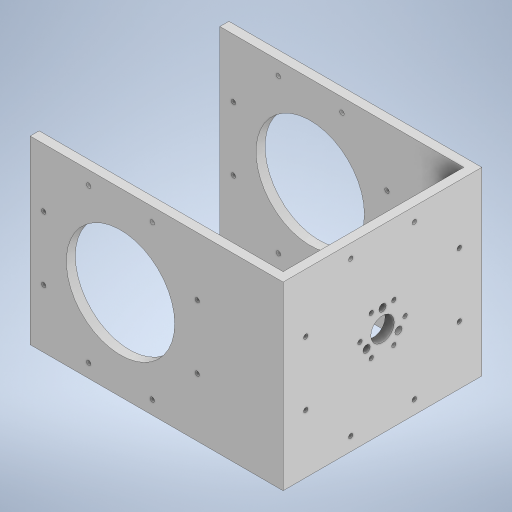
# Autodesk Inventor part: legparts_07(three)
Saved by Autodesk Inventor 2024.3 (Build 283343000, 343)
## iProperties
Created: 2024-10-21
Part Number: legparts_07(three)
Material: 一般
Document SubType Name: Modeling
Designer: 佐藤智貴
Density: 1 g/cm^3
Appearance: 既定
Mass: 104.488 g
Surface Area: 473.803 cm^2
Volume: 104.488 cm^3
Author: 佐藤智貴
Autodesk Inventor part; units mm, degrees
ref_plane "YZ Plane" through (0, 0, 0) normal (1, 0, 0) x (0, 1, 0)
ref_plane "XZ Plane" through (0, 0, 0) normal (0, 1, 0) x (-1, 0, 0)
ref_plane "XY Plane" through (0, 0, 0) normal (0, 0, 1) x (1, 0, 0)
sketch "スケッチ1" plane through (0, 0, 0) normal (0, 0, 1) x (1, 0, 0)
  circle A0 centre (0, 0) radius 48.5
  circle A1 centre (0, 0) radius 46.0893
  line L0 (-50, 50) -> (50, 50)
  line L1 (50, 50) -> (50, -50)
  line L2 (50, -50) -> (-50, -50)
  line L3 (-50, -50) -> (-50, 50)
  dimension "d0" = 97
  dimension "d3" = 50
  dimension "d4" = 50
  dimension "d5" = 50
  dimension "d6" = 50
  constraints: 8 end point, 2 centre point, 2 parallel, 1 coincident, 1 horizontal, 1 perpendicular
  measures "d0" diameter of A0
  measures "d3" distance from line of L0 point (0, 0)
  measures "d4" distance from line of L2 point (0, 0)
  measures "d5" distance from line of L1 point (0, 0)
  measures "d6" distance from line of point (0, 0) L3
extrude "押し出し1" add sketch "スケッチ1" along normal blind 5 contours A0 | A1 | L0 L1 L2 L3
sketch "スケッチ2" plane through (0, 0, 5) normal (0, 0, 1) x (1, 0, 0)
  circle A0 centre (0, 0) radius 46
  line L0 (0, 0) -> (0, 64.6511)
  line L1 (0, 0) -> (-25.9524, 62.6547)
  line L2 (-50, 50) -> (-50, -50) projected
  point P0 (-17.6034, 42.4985)
  point P1 (-42.4985, 17.6034)
  point P2 (-42.4985, -17.6034)
  point P3 (-17.6034, -42.4985)
  point P4 (17.6034, -42.4985)
  point P5 (42.4985, -17.6034)
  point P6 (42.4985, 17.6034)
  point P7 (17.6034, 42.4985)
  dimension "d7" = 92
  dimension "d8" = 22.5
  dimension "d11" = 360
  dimension "d76" = 50
  constraints: 4 end point, 1 coincident, 1 point on line, 1 vertical, 12 other
  measures "d8" angle of L0 L1
  measures "d76" distance from line of L2 point (0, 0)
hole "穴1" at (-17.6034, 42.4985, 5) at (-42.4985, 17.6034, 5) at (-42.4985, -17.6034, 5) at (-17.6034, -42.4985, 5) at (17.6034, -42.4985, 5) at (42.4985, -17.6034, 5) at (42.4985, 17.6034, 5) at (17.6034, 42.4985, 5) direction (0, 0, -1) diameter 2.459 end through all
sketch "スケッチ3" plane through (0, 0, 5) normal (0, 0, 1) x (1, 0, 0)
  circle A0 centre (0, 0) radius 30
  dimension "d20" = 60
  constraints: 1 centre point, 1 coincident
  measures "d20" diameter of A0
extrude "押し出し2" cut sketch "スケッチ3" against normal blind 5
sketch "スケッチ4" plane through (50, -50, 0) normal (1, 0, 0) x (0, 0, -1)
  line L0 (-5, 100) -> (-5, 0) projected
  line L1 (-5, 100) -> (0, 100)
  line L2 (0, 100) -> (0, 0)
  line L3 (0, 0) -> (-5, 0)
  line L4 (-5, 0) -> (-5, 100)
  point P0 (0, 50)
  constraints: 8 end point, 2 parallel, 1 horizontal, 1 perpendicular
extrude "押し出し3" add sketch "スケッチ4" along normal blind 40
sketch "スケッチ5" plane through (0, 0, 5) normal (0, 0, 1) x (1, 0, 0)
  line L0 (-50, 50) -> (90, 50) projected
  line L1 (85, 50) -> (90, 50)
  line L2 (90, 50) -> (90, -50)
  line L3 (90, -50) -> (85, -50)
  line L4 (85, -50) -> (85, 50)
  line L5 (-50, -50) -> (90, -50) projected
  line L6 (90, 50) -> (90, -50) projected
  point P0 (0, 0)
  point P1 (90, 50)
  point P2 (90, 0)
  dimension "d25" = 0
  dimension "d26" = 5
  dimension "d27" = 100
  dimension "d70" = 0
  constraints: 8 end point, 2 parallel, 1 horizontal, 1 midpoint, 1 perpendicular, 1 point on line
  measures "d25" distance from line of L5 L2.end
  measures "d26" distance between parallel lines of L2 L4
  measures "d27" distance of L1.end L2.end
  measures "d70" distance from line of L6 point (90, 0)
extrude "押し出し4" add sketch "スケッチ5" along normal blind 100
sketch "スケッチ6" plane through (90, -50, 0) normal (1, 0, 0) x (0, 0, -1)
  circle A0 centre (-55, 50) radius 46
  line L0 (0, 0) -> (-105, 0) projected
  line L1 (0, 0) -> (0, 100) projected
  line L2 (-55, 50) -> (41.9537, 50)
  line L3 (-55, 50) -> (-55, 131.7305)
  line L4 (-55, 50) -> (-80.0101, 110.3797)
  circle A1 centre (-55, 50) radius 12.5
  line L5 (-55, 50) -> (-63.1841, 64.1753)
  point P0 (0, 50)
  point P1 (-72.6034, 92.4985)
  point P2 (-97.4985, 67.6034)
  point P3 (-97.4985, 32.3966)
  point P4 (-72.6034, 7.5015)
  point P5 (-37.3966, 7.5015)
  point P6 (-12.5015, 32.3966)
  point P7 (-12.5015, 67.6034)
  point P8 (-37.3966, 92.4985)
  point P9 (-61.25, 60.8253)
  point P10 (-67.5, 50)
  point P11 (-61.25, 39.1747)
  point P12 (-48.75, 39.1747)
  point P13 (-42.5, 50)
  point P14 (-48.75, 60.8253)
  dimension "d32" = 92
  dimension "d34" = 25
  dimension "d30" = 50
  dimension "d31" = 55
  dimension "d33" = 22.5
  dimension "d35" = 30
  dimension "d38" = 360
  dimension "d42" = 360
  constraints: 8 end point, 2 point on line, 1 coincident, 1 horizontal, 1 vertical, 22 other
  measures "d30" distance from line of L0 L2.start
  measures "d31" distance from line of L1 L2.start
  measures "d33" angle of L4 L3
  measures "d35" angle of L3 L5
hole "穴2" at (90, 42.4985, 72.6034) at (90, 17.6034, 97.4985) at (90, -17.6034, 97.4985) at (90, -42.4985, 72.6034) at (90, -42.4985, 37.3966) at (90, -17.6034, 12.5015) at (90, 17.6034, 12.5015) at (90, 42.4985, 37.3966) at (90, 10.8253, 61.25) at (90, 0, 67.5) at (90, -10.8253, 61.25) at (90, -10.8253, 48.75) at (90, 0, 42.5) at (90, 10.8253, 48.75) direction (-1, 0, 0) diameter 2.459 end through all
sketch "スケッチ7" plane through (90, -50, 0) normal (1, 0, 0) x (0, 0, -1)
  line L0 (-55, 50) -> (26.223, 50)
  circle A0 centre (-55, 50) radius 10.2
  line L1 (0, 0) -> (0, 100) projected
  line L2 (0, 0) -> (-105, 0) projected
  line L3 (-55, 50) -> (-55, 82.0983)
  point P0 (0, 50)
  point P1 (-55, 60.2)
  point P2 (-63.8335, 44.9)
  point P3 (-46.1665, 44.9)
  dimension "d53" = 20.4
  dimension "d51" = 55
  dimension "d52" = 50
  dimension "d56" = 360
  constraints: 4 end point, 1 coincident, 1 horizontal, 1 point on line, 1 vertical, 1 vertical alignment, 6 other
  measures "d51" distance from line of L1 L3.start
  measures "d52" distance from line of L2 L3.start
hole "穴3" at (90, 10.2, 55) at (90, -5.1, 63.8335) at (90, -5.1, 46.1665) direction (-1, 0, 0) diameter 4 end through all
sketch "スケッチ8" plane through (90, -50, 0) normal (1, 0, 0) x (0, 0, -1)
  circle A0 centre (-55, 50) radius 6.5
  line L0 (0, 0) -> (0, 100) projected
  line L1 (0, 0) -> (-105, 0) projected
  point P0 (0, 50)
  dimension "d65" = 13
  dimension "d66" = 55
  dimension "d67" = 50
  constraints: 1 centre point
  measures "d65" diameter of A0
  measures "d66" distance from line of L0 A0.centre
  measures "d67" distance from line of L1 A0.centre
extrude "押し出し5" cut sketch "スケッチ8" against normal through all
sketch "スケッチ9" plane through (0, 0, 105) normal (0, 0, 1) x (1, 0, 0)
  line L0 (-50, 50) -> (85, 50) projected
  line L1 (-50, -50) -> (90, -50) projected
  line L2 (85, 50) -> (90, 50)
  line L3 (90, 50) -> (90, -50)
  line L4 (90, -50) -> (85, -50)
  line L5 (85, -50) -> (85, 50)
  point P0 (0, 0)
  constraints: 8 end point, 2 parallel, 1 horizontal, 1 perpendicular
extrude "押し出し6" add sketch "スケッチ9" along normal blind 5
sketch "スケッチ10" plane through (85, -50, 5) normal (-1, 0, 0) x (0, 0, 1)
  line L0 (105, 100) -> (105, 0) projected
  line L1 (-5, 0) -> (105, 0) projected
  line L2 (105, 100) -> (100, 100)
  line L3 (100, 100) -> (100, 0)
  line L4 (100, 0) -> (105, 0)
  line L5 (105, 0) -> (105, 100)
  point P0 (-5, 50)
  dimension "d73" = 5
  constraints: 8 end point, 2 parallel, 1 horizontal, 1 perpendicular, 1 point on line
  measures "d73" distance between parallel lines of L0 L3
extrude "押し出し7" add sketch "スケッチ10" along normal blind 135
sketch "スケッチ11" plane through (0, 0, 110) normal (0, 0, 1) x (1, 0, 0)
  circle A0 centre (0, 0) radius 46
  line L0 (0, 0) -> (0, 49.674)
  line L1 (0, 0) -> (-20.8641, 50.3704)
  point P0 (-17.6034, 42.4985)
  point P1 (-42.4985, 17.6034)
  point P2 (-42.4985, -17.6034)
  point P3 (-17.6034, -42.4985)
  point P4 (17.6034, -42.4985)
  point P5 (42.4985, -17.6034)
  point P6 (42.4985, 17.6034)
  point P7 (17.6034, 42.4985)
  dimension "d79" = 92
  dimension "d80" = 22.5
  dimension "d81" = 360
  constraints: 4 end point, 2 coincident, 1 point on line, 1 vertical, 12 other
  measures "d80" angle of L0 L1
hole "穴4" at (-17.6034, 42.4985, 110) at (17.6034, 42.4985, 110) at (42.4985, 17.6034, 110) at (42.4985, -17.6034, 110) at (17.6034, -42.4985, 110) at (-17.6034, -42.4985, 110) at (-42.4985, -17.6034, 110) at (-42.4985, 17.6034, 110) direction (0, 0, -1) diameter 2.459 end through all
sketch "スケッチ12" plane through (0, 0, 110) normal (0, 0, 1) x (1, 0, 0)
  circle A0 centre (0, 0) radius 30 projected
  circle A1 centre (0, 0) radius 30
  constraints: 1 centre point, 1 coincident
extrude "押し出し8" cut sketch "スケッチ12" against normal blind 135
equation "\"d4\" = d3"
equation "\"d5\" = d3"
equation "\"d6\" = d5"
